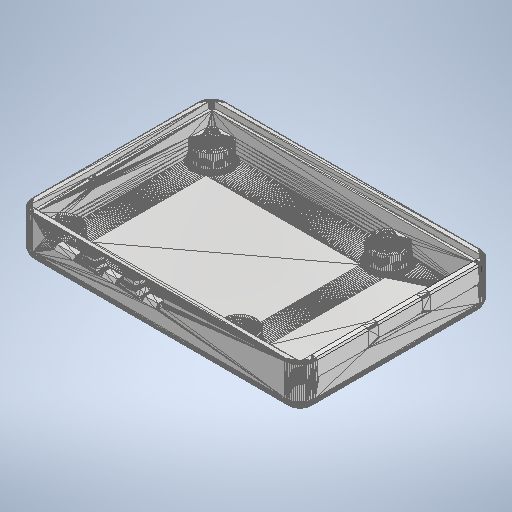
# Autodesk Inventor part: base_01
Saved by Autodesk Inventor 2025.2 (Build 292293000, 293)
## iProperties
Created: 2026-02-21
Part Number: base_01
Material: 一般
Document SubType Name: Modeling
Designer: naka6
Density: 1 g/cm^3
Appearance: 既定
Author: naka6
Autodesk Inventor part; units mm, degrees
ref_plane "YZ Plane" through (0, 0, 0) normal (1, 0, 0) x (0, 1, 0)
ref_plane "XZ Plane" through (0, 0, 0) normal (0, 1, 0) x (-1, 0, 0)
ref_plane "XY Plane" through (0, 0, 0) normal (0, 0, 1) x (1, 0, 0)
sketch "スケッチ1" plane through (43.5, 1.6, 26.25) normal (0, 0, -1) x (-1, 0, 0)
  line L0 (-3, 0.5001) -> (-3, -0.5) projected
  line L1 (0, -0.5) -> (0, 0.4999) projected
  line L2 (0, -0.0868) -> (0, 2.9) projected
  line L3 (-3, -0.0868) -> (-3, 4.4) projected
  circle A0 centre (-3, 4.9) radius 0.5 projected
  line L4 (-1, 4.9) -> (-2.5, 4.9) projected
  line L5 (-1, 4.9) -> (-0.9302, 2.9) projected
  line L6 (-0.9302, 2.9) -> (0, 2.9) projected
  line L7 (-3, -0.5) -> (0, -0.5)
  point P0 (43.5, -1.6)
  point P1 (-2.5, 4.9)
  constraints: 2 end point, 1 other
extrude "押し出し1" add sketch "スケッチ1" along normal blind 54 contours L3 A0 L4 L5 L6 L2 L1 L7 L0
